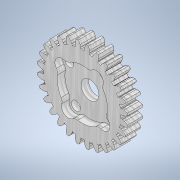
# Autodesk Inventor part: m1歯数28ギア5td6
Saved by Autodesk Inventor 2020.2 (Build 242310000, 310)
## iProperties
Created: 2020-02-29
Part Number: m1歯数28ギア5td6
Material: アルミニウム 7075
Document SubType Name: Modeling
Designer: aoyam
Density: 2.81 g/cm^3
Appearance: サテン - ブラシ仕上げ 重厚
Author: aoyam
Autodesk Inventor part; units mm, degrees
ref_plane "YZ Plane" through (0, 0, 0) normal (1, 0, 0) x (0, 1, 0)
ref_plane "XZ Plane" through (0, 0, 0) normal (0, 1, 0) x (-1, 0, 0)
ref_plane "XY Plane" through (0, 0, 0) normal (0, 0, 1) x (1, 0, 0)
sketch "スケッチ1" plane through (0, 0, 0) normal (0, 0, 1) x (1, 0, 0)
  arc A0 (-2.9821, 27.222) -> (-3.0107, 27.0374) centre (-1.7695, 26.9398) ccw
  arc A1 (-2.798, 27.798) -> (-2.9821, 27.222) centre (0.3539, 26.4732) ccw
  arc A2 (-2.2367, 28.835) -> (-2.798, 27.798) centre (2.6408, 25.5245) ccw
  arc A3 (-4.0943, 27.0374) -> (-4.1229, 27.222) centre (-5.3355, 26.9398) ccw
  arc A4 (-4.1229, 27.222) -> (-4.307, 27.798) centre (-7.4589, 26.4732) ccw
  arc A5 (-4.307, 27.798) -> (-4.8683, 28.835) centre (-9.7458, 25.5245) ccw
  arc A6 (-3.0274, 26.632) -> (-4.0776, 26.632) centre (-3.5525, 13.8928) ccw
  arc A7 (-4.8683, 28.835) -> (-5.5946, 28.7532) centre (-3.5525, 13.8928) ccw
  line L0 (-3.0274, 26.632) -> (-3.0107, 27.0374)
  line L1 (-4.0776, 26.632) -> (-4.0943, 27.0374)
  line L2 (-6.8991, 26.1958) -> (-7.0056, 26.5873)
  arc A8 (-7.0056, 26.5873) -> (-7.0746, 26.7609) centre (-8.194, 26.2159) ccw
  arc A9 (-7.0746, 26.7609) -> (-7.3822, 27.2815) centre (-10.1603, 25.2886) ccw
  arc A10 (-7.3822, 27.2815) -> (-8.1602, 28.1676) centre (-12.1788, 23.8547) ccw
  arc A11 (-8.1602, 28.1676) -> (-8.8502, 27.9262) centre (-3.5525, 13.8928) ccw
  arc A12 (-5.8753, 26.4295) -> (-6.8991, 26.1958) centre (-3.5525, 13.8928) ccw
  line L3 (-5.8753, 26.4295) -> (-5.9492, 26.8284)
  arc A13 (-5.9624, 27.0148) -> (-5.9492, 26.8284) centre (-4.7174, 27.0094) ccw
  arc A14 (-5.9111, 27.6173) -> (-5.9624, 27.0148) centre (-2.5434, 27.0271) ccw
  arc A15 (-5.5946, 28.7532) -> (-5.9111, 27.6173) centre (-0.1027, 26.611) ccw
  line L4 (-9.5529, 25.1426) -> (-9.7438, 25.5006)
  arc A16 (-9.7438, 25.5006) -> (-9.8497, 25.6546) centre (-10.8197, 24.8741) ccw
  arc A17 (-9.8497, 25.6546) -> (-10.2655, 26.0936) centre (-12.5304, 23.5325) ccw
  arc A18 (-10.2655, 26.0936) -> (-11.2211, 26.7844) centre (-14.1792, 21.6854) ccw
  arc A19 (-11.2211, 26.7844) -> (-11.84, 26.3955) centre (-3.5525, 13.8928) ccw
  arc A20 (-8.6067, 25.5983) -> (-9.5529, 25.1426) centre (-3.5525, 13.8928) ccw
  line L5 (-8.6067, 25.5983) -> (-8.7675, 25.9707)
  arc A21 (-8.8219, 26.1495) -> (-8.7675, 25.9707) centre (-7.6069, 26.4213) ccw
  arc A22 (-8.9059, 26.7483) -> (-8.8219, 26.1495) centre (-5.4914, 26.9223) ccw
  arc A23 (-8.8502, 27.9262) -> (-8.9059, 26.7483) centre (-3.0193, 27.0598) ccw
  line L6 (-11.9058, 23.5254) -> (-12.1716, 23.8319)
  arc A24 (-12.1716, 23.8319) -> (-12.309, 23.9584) centre (-13.0811, 22.9817) ccw
  arc A25 (-12.309, 23.9584) -> (-12.8121, 24.2939) centre (-14.4504, 21.293) ccw
  arc A26 (-12.8121, 24.2939) -> (-13.8975, 24.7547) centre (-15.6468, 19.1254) ccw
  arc A27 (-13.8975, 24.7547) -> (-14.4144, 24.2379) centre (-3.5525, 13.8928) ccw
  arc A28 (-11.0847, 24.1801) -> (-11.9058, 23.5254) centre (-3.5525, 13.8928) ccw
  line L7 (-11.0847, 24.1801) -> (-11.3244, 24.5075)
  arc A29 (-11.4171, 24.6697) -> (-11.3244, 24.5075) centre (-10.2931, 25.205) ccw
  arc A30 (-11.6323, 25.2347) -> (-11.4171, 24.6697) centre (-8.3421, 26.1642) ccw
  arc A31 (-11.84, 26.3955) -> (-11.6323, 25.2347) centre (-5.9626, 26.8483) ccw
  line L8 (-13.8398, 21.4251) -> (-14.1671, 21.6647)
  arc A32 (-14.1671, 21.6647) -> (-14.3293, 21.7575) centre (-14.8646, 20.6335) ccw
  arc A33 (-14.3293, 21.7575) -> (-14.8944, 21.9727) centre (-15.8238, 18.6824) ccw
  arc A34 (-14.8944, 21.9727) -> (-16.0551, 22.1804) centre (-16.5079, 16.3029) ccw
  arc A35 (-16.0551, 22.1804) -> (-16.444, 21.5615) centre (-3.5525, 13.8928) ccw
  arc A36 (-13.185, 22.2461) -> (-13.8398, 21.4251) centre (-3.5525, 13.8928) ccw
  line L9 (-13.185, 22.2461) -> (-13.4915, 22.5119)
  arc A37 (-13.618, 22.6494) -> (-13.4915, 22.5119) centre (-12.6413, 23.4214) ccw
  arc A38 (-13.9536, 23.1524) -> (-13.618, 22.6494) centre (-10.9526, 24.7907) ccw
  arc A39 (-14.4144, 24.2379) -> (-13.9536, 23.1524) centre (-8.785, 25.9872) ccw
  line L10 (-15.2579, 18.9471) -> (-15.6304, 19.1079)
  arc A40 (-15.6304, 19.1079) -> (-15.8092, 19.1623) centre (-16.0809, 17.9473) ccw
  arc A41 (-15.8092, 19.1623) -> (-16.4079, 19.2463) centre (-16.5819, 15.8317) ccw
  arc A42 (-16.4079, 19.2463) -> (-17.5858, 19.1905) centre (-16.7194, 13.3597) ccw
  arc A43 (-17.5858, 19.1905) -> (-17.8272, 18.5006) centre (-3.5525, 13.8928) ccw
  arc A44 (-14.8023, 19.8933) -> (-15.2579, 18.9471) centre (-3.5525, 13.8928) ccw
  line L11 (-14.8023, 19.8933) -> (-15.1602, 20.0842)
  arc A45 (-15.3142, 20.1901) -> (-15.1602, 20.0842) centre (-14.5337, 21.1601) ccw
  arc A46 (-15.7532, 20.6058) -> (-15.3142, 20.1901) centre (-13.1921, 22.8708) ccw
  arc A47 (-16.444, 21.5615) -> (-15.7532, 20.6058) centre (-11.3451, 24.5196) ccw
  line L12 (-16.0891, 16.2157) -> (-16.488, 16.2896)
  arc A48 (-16.488, 16.2896) -> (-16.6744, 16.3028) centre (-16.669, 15.0578) ccw
  arc A49 (-16.6744, 16.3028) -> (-17.2769, 16.2515) centre (-16.6867, 12.8838) ccw
  arc A50 (-17.2769, 16.2515) -> (-18.4128, 15.935) centre (-16.2707, 10.4431) ccw
  arc A51 (-18.4128, 15.935) -> (-18.4947, 15.2086) centre (-3.5525, 13.8928) ccw
  arc A52 (-15.8554, 17.2395) -> (-16.0891, 16.2157) centre (-3.5525, 13.8928) ccw
  line L13 (-15.8554, 17.2395) -> (-16.2469, 17.346)
  arc A53 (-16.4206, 17.415) -> (-16.2469, 17.346) centre (-15.8755, 18.5343) ccw
  arc A54 (-16.9411, 17.7226) -> (-16.4206, 17.415) centre (-14.9482, 20.5007) ccw
  arc A55 (-17.8272, 18.5006) -> (-16.9411, 17.7226) centre (-13.5144, 22.5192) ccw
  line L14 (-16.2917, 13.3678) -> (-16.697, 13.351)
  arc A56 (-16.697, 13.351) -> (-16.8817, 13.3225) centre (-16.5994, 12.1099) ccw
  arc A57 (-16.8817, 13.3225) -> (-17.4576, 13.1384) centre (-16.1329, 9.9864) ccw
  arc A58 (-17.4576, 13.1384) -> (-18.4947, 12.5771) centre (-15.1841, 7.6995) ccw
  arc A59 (-18.4947, 12.5771) -> (-18.4128, 11.8507) centre (-3.5525, 13.8928) ccw
  arc A60 (-16.2917, 14.4179) -> (-16.2917, 13.3678) centre (-3.5525, 13.8928) ccw
  line L15 (-16.2917, 14.4179) -> (-16.697, 14.4346)
  arc A61 (-16.8817, 14.4632) -> (-16.697, 14.4346) centre (-16.5994, 15.6758) ccw
  arc A62 (-17.4576, 14.6473) -> (-16.8817, 14.4632) centre (-16.1329, 17.7992) ccw
  arc A63 (-18.4947, 15.2086) -> (-17.4576, 14.6473) centre (-15.1841, 20.0862) ccw
  line L16 (-15.8554, 10.5462) -> (-16.2469, 10.4397)
  arc A64 (-16.2469, 10.4397) -> (-16.4206, 10.3707) centre (-15.8755, 9.2514) ccw
  arc A65 (-16.4206, 10.3707) -> (-16.9411, 10.0631) centre (-14.9482, 7.285) ccw
  arc A66 (-16.9411, 10.0631) -> (-17.8272, 9.2851) centre (-13.5144, 5.2665) ccw
  arc A67 (-17.8272, 9.2851) -> (-17.5858, 8.5952) centre (-3.5525, 13.8928) ccw
  arc A68 (-16.0891, 11.57) -> (-15.8554, 10.5462) centre (-3.5525, 13.8928) ccw
  line L17 (-16.0891, 11.57) -> (-16.488, 11.4961)
  arc A69 (-16.6744, 11.4829) -> (-16.488, 11.4961) centre (-16.669, 12.7279) ccw
  arc A70 (-17.2769, 11.5342) -> (-16.6744, 11.4829) centre (-16.6867, 14.9019) ccw
  arc A71 (-18.4128, 11.8507) -> (-17.2769, 11.5342) centre (-16.2707, 17.3426) ccw
  line L18 (-14.8023, 7.8924) -> (-15.1602, 7.7015)
  arc A72 (-15.1602, 7.7015) -> (-15.3142, 7.5956) centre (-14.5337, 6.6256) ccw
  arc A73 (-15.3142, 7.5956) -> (-15.7532, 7.1799) centre (-13.1921, 4.9149) ccw
  arc A74 (-15.7532, 7.1799) -> (-16.444, 6.2242) centre (-11.3451, 3.2661) ccw
  arc A75 (-16.444, 6.2242) -> (-16.0551, 5.6053) centre (-3.5525, 13.8928) ccw
  arc A76 (-15.2579, 8.8386) -> (-14.8023, 7.8924) centre (-3.5525, 13.8928) ccw
  line L19 (-15.2579, 8.8386) -> (-15.6304, 8.6778)
  arc A77 (-15.8092, 8.6234) -> (-15.6304, 8.6778) centre (-16.0809, 9.8384) ccw
  arc A78 (-16.4079, 8.5394) -> (-15.8092, 8.6234) centre (-16.5819, 11.954) ccw
  arc A79 (-17.5858, 8.5952) -> (-16.4079, 8.5394) centre (-16.7194, 14.426) ccw
  line L20 (-13.185, 5.5396) -> (-13.4915, 5.2738)
  arc A80 (-13.4915, 5.2738) -> (-13.618, 5.1363) centre (-12.6413, 4.3642) ccw
  arc A81 (-13.618, 5.1363) -> (-13.9536, 4.6333) centre (-10.9526, 2.995) ccw
  arc A82 (-13.9536, 4.6333) -> (-14.4144, 3.5478) centre (-8.785, 1.7985) ccw
  arc A83 (-14.4144, 3.5478) -> (-13.8975, 3.031) centre (-3.5525, 13.8928) ccw
  arc A84 (-13.8398, 6.3606) -> (-13.185, 5.5396) centre (-3.5525, 13.8928) ccw
  line L21 (-13.8398, 6.3606) -> (-14.1671, 6.121)
  arc A85 (-14.3293, 6.0282) -> (-14.1671, 6.121) centre (-14.8646, 7.1522) ccw
  arc A86 (-14.8944, 5.813) -> (-14.3293, 6.0282) centre (-15.8238, 9.1033) ccw
  arc A87 (-16.0551, 5.6053) -> (-14.8944, 5.813) centre (-16.5079, 11.4827) ccw
  line L22 (-11.0847, 3.6056) -> (-11.3244, 3.2782)
  arc A88 (-11.3244, 3.2782) -> (-11.4171, 3.116) centre (-10.2931, 2.5807) ccw
  arc A89 (-11.4171, 3.116) -> (-11.6323, 2.551) centre (-8.3421, 1.6215) ccw
  arc A90 (-11.6323, 2.551) -> (-11.84, 1.3902) centre (-5.9626, 0.9374) ccw
  arc A91 (-11.84, 1.3902) -> (-11.2211, 1.0013) centre (-3.5525, 13.8928) ccw
  arc A92 (-11.9058, 4.2603) -> (-11.0847, 3.6056) centre (-3.5525, 13.8928) ccw
  line L23 (-11.9058, 4.2603) -> (-12.1716, 3.9538)
  arc A93 (-12.309, 3.8273) -> (-12.1716, 3.9538) centre (-13.0811, 4.804) ccw
  arc A94 (-12.8121, 3.4918) -> (-12.309, 3.8273) centre (-14.4504, 6.4927) ccw
  arc A95 (-13.8975, 3.031) -> (-12.8121, 3.4918) centre (-15.6468, 8.6603) ccw
  line L24 (-8.6067, 2.1874) -> (-8.7675, 1.815)
  arc A96 (-8.7675, 1.815) -> (-8.8219, 1.6362) centre (-7.6069, 1.3644) ccw
  arc A97 (-8.8219, 1.6362) -> (-8.9059, 1.0374) centre (-5.4914, 0.8634) ccw
  arc A98 (-8.9059, 1.0374) -> (-8.8502, -0.1405) centre (-3.0193, 0.7259) ccw
  arc A99 (-8.8502, -0.1405) -> (-8.1602, -0.3819) centre (-3.5525, 13.8928) ccw
  arc A100 (-9.5529, 2.6431) -> (-8.6067, 2.1874) centre (-3.5525, 13.8928) ccw
  line L25 (-9.5529, 2.6431) -> (-9.7438, 2.2851)
  arc A101 (-9.8497, 2.1311) -> (-9.7438, 2.2851) centre (-10.8197, 2.9116) ccw
  arc A102 (-10.2655, 1.6921) -> (-9.8497, 2.1311) centre (-12.5304, 4.2532) ccw
  arc A103 (-11.2211, 1.0013) -> (-10.2655, 1.6921) centre (-14.1792, 6.1003) ccw
  line L26 (-5.8753, 1.3562) -> (-5.9492, 0.9573)
  arc A104 (-5.9492, 0.9573) -> (-5.9624, 0.7709) centre (-4.7174, 0.7763) ccw
  arc A105 (-5.9624, 0.7709) -> (-5.9111, 0.1684) centre (-2.5434, 0.7586) ccw
  arc A106 (-5.9111, 0.1684) -> (-5.5946, -0.9675) centre (-0.1027, 1.1747) ccw
  arc A107 (-5.5946, -0.9675) -> (-4.8683, -1.0493) centre (-3.5525, 13.8928) ccw
  arc A108 (-6.8991, 1.5899) -> (-5.8753, 1.3562) centre (-3.5525, 13.8928) ccw
  line L27 (-6.8991, 1.5899) -> (-7.0056, 1.1984)
  arc A109 (-7.0746, 1.0248) -> (-7.0056, 1.1984) centre (-8.194, 1.5698) ccw
  arc A110 (-7.3822, 0.5042) -> (-7.0746, 1.0248) centre (-10.1603, 2.4971) ccw
  arc A111 (-8.1602, -0.3819) -> (-7.3822, 0.5042) centre (-12.1788, 3.931) ccw
  line L28 (-3.0274, 1.1537) -> (-3.0107, 0.7483)
  arc A112 (-3.0107, 0.7483) -> (-2.9821, 0.5637) centre (-1.7695, 0.8459) ccw
  arc A113 (-2.9821, 0.5637) -> (-2.798, -0.0123) centre (0.3539, 1.3125) ccw
  arc A114 (-2.798, -0.0123) -> (-2.2367, -1.0493) centre (2.6408, 2.2612) ccw
  arc A115 (-2.2367, -1.0493) -> (-1.5103, -0.9675) centre (-3.5525, 13.8928) ccw
  arc A116 (-4.0776, 1.1537) -> (-3.0274, 1.1537) centre (-3.5525, 13.8928) ccw
  line L29 (-4.0776, 1.1537) -> (-4.0943, 0.7483)
  arc A117 (-4.1229, 0.5637) -> (-4.0943, 0.7483) centre (-5.3355, 0.8459) ccw
  arc A118 (-4.307, -0.0123) -> (-4.1229, 0.5637) centre (-7.4589, 1.3125) ccw
  arc A119 (-4.8683, -1.0493) -> (-4.307, -0.0123) centre (-9.7458, 2.2612) ccw
  line L30 (-0.2058, 1.5899) -> (-0.0993, 1.1984)
  arc A120 (-0.0993, 1.1984) -> (-0.0304, 1.0248) centre (1.089, 1.5698) ccw
  arc A121 (-0.0304, 1.0248) -> (0.2773, 0.5042) centre (3.0554, 2.4971) ccw
  arc A122 (0.2773, 0.5042) -> (1.0553, -0.3819) centre (5.0738, 3.931) ccw
  arc A123 (1.0553, -0.3819) -> (1.7452, -0.1405) centre (-3.5525, 13.8928) ccw
  arc A124 (-1.2297, 1.3562) -> (-0.2058, 1.5899) centre (-3.5525, 13.8928) ccw
  line L31 (-1.2297, 1.3562) -> (-1.1558, 0.9573)
  arc A125 (-1.1425, 0.7709) -> (-1.1558, 0.9573) centre (-2.3875, 0.7763) ccw
  arc A126 (-1.1938, 0.1684) -> (-1.1425, 0.7709) centre (-4.5615, 0.7586) ccw
  arc A127 (-1.5103, -0.9675) -> (-1.1938, 0.1684) centre (-7.0022, 1.1747) ccw
  line L32 (2.4479, 2.6431) -> (2.6389, 2.2851)
  arc A128 (2.6389, 2.2851) -> (2.7447, 2.1311) centre (3.7148, 2.9116) ccw
  arc A129 (2.7447, 2.1311) -> (3.1605, 1.6921) centre (5.4255, 4.2532) ccw
  arc A130 (3.1605, 1.6921) -> (4.1162, 1.0013) centre (7.0743, 6.1003) ccw
  arc A131 (4.1162, 1.0013) -> (4.7351, 1.3902) centre (-3.5525, 13.8928) ccw
  arc A132 (1.5018, 2.1874) -> (2.4479, 2.6431) centre (-3.5525, 13.8928) ccw
  line L33 (1.5018, 2.1874) -> (1.6626, 1.815)
  arc A133 (1.7169, 1.6362) -> (1.6626, 1.815) centre (0.502, 1.3644) ccw
  arc A134 (1.801, 1.0374) -> (1.7169, 1.6362) centre (-1.6136, 0.8634) ccw
  arc A135 (1.7452, -0.1405) -> (1.801, 1.0374) centre (-4.0857, 0.7259) ccw
  line L34 (4.8008, 4.2603) -> (5.0666, 3.9538)
  arc A136 (5.0666, 3.9538) -> (5.2041, 3.8273) centre (5.9761, 4.804) ccw
  arc A137 (5.2041, 3.8273) -> (5.7071, 3.4918) centre (7.3454, 6.4927) ccw
  arc A138 (5.7071, 3.4918) -> (6.7925, 3.031) centre (8.5419, 8.6603) ccw
  arc A139 (6.7925, 3.031) -> (7.3094, 3.5478) centre (-3.5525, 13.8928) ccw
  arc A140 (3.9797, 3.6056) -> (4.8008, 4.2603) centre (-3.5525, 13.8928) ccw
  line L35 (3.9797, 3.6056) -> (4.2194, 3.2782)
  arc A141 (4.3122, 3.116) -> (4.2194, 3.2782) centre (3.1881, 2.5807) ccw
  arc A142 (4.5274, 2.551) -> (4.3122, 3.116) centre (1.2371, 1.6215) ccw
  arc A143 (4.7351, 1.3902) -> (4.5274, 2.551) centre (-1.1424, 0.9374) ccw
  line L36 (6.7348, 6.3606) -> (7.0621, 6.121)
  arc A144 (7.0621, 6.121) -> (7.2243, 6.0282) centre (7.7597, 7.1522) ccw
  arc A145 (7.2243, 6.0282) -> (7.7894, 5.813) centre (8.7189, 9.1033) ccw
  arc A146 (7.7894, 5.813) -> (8.9502, 5.6053) centre (9.403, 11.4827) ccw
  arc A147 (8.9502, 5.6053) -> (9.3391, 6.2242) centre (-3.5525, 13.8928) ccw
  arc A148 (6.08, 5.5396) -> (6.7348, 6.3606) centre (-3.5525, 13.8928) ccw
  line L37 (6.08, 5.5396) -> (6.3865, 5.2738)
  arc A149 (6.5131, 5.1363) -> (6.3865, 5.2738) centre (5.5363, 4.3642) ccw
  arc A150 (6.8486, 4.6333) -> (6.5131, 5.1363) centre (3.8477, 2.995) ccw
  arc A151 (7.3094, 3.5478) -> (6.8486, 4.6333) centre (1.6801, 1.7985) ccw
  line L38 (8.153, 8.8386) -> (8.5254, 8.6778)
  arc A152 (8.5254, 8.6778) -> (8.7042, 8.6234) centre (8.976, 9.8384) ccw
  arc A153 (8.7042, 8.6234) -> (9.303, 8.5394) centre (9.477, 11.954) ccw
  arc A154 (9.303, 8.5394) -> (10.4809, 8.5952) centre (9.6145, 14.426) ccw
  arc A155 (10.4809, 8.5952) -> (10.7223, 9.2851) centre (-3.5525, 13.8928) ccw
  arc A156 (7.6973, 7.8924) -> (8.153, 8.8386) centre (-3.5525, 13.8928) ccw
  line L39 (7.6973, 7.8924) -> (8.0553, 7.7015)
  arc A157 (8.2092, 7.5956) -> (8.0553, 7.7015) centre (7.4288, 6.6256) ccw
  arc A158 (8.6483, 7.1799) -> (8.2092, 7.5956) centre (6.0871, 4.9149) ccw
  arc A159 (9.3391, 6.2242) -> (8.6483, 7.1799) centre (4.2401, 3.2661) ccw
  line L40 (8.9841, 11.57) -> (9.3831, 11.4961)
  arc A160 (9.3831, 11.4961) -> (9.5694, 11.4829) centre (9.5641, 12.7279) ccw
  arc A161 (9.5694, 11.4829) -> (10.1719, 11.5342) centre (9.5817, 14.9019) ccw
  arc A162 (10.1719, 11.5342) -> (11.3079, 11.8507) centre (9.1657, 17.3426) ccw
  arc A163 (11.3079, 11.8507) -> (11.3897, 12.5771) centre (-3.5525, 13.8928) ccw
  arc A164 (8.7505, 10.5462) -> (8.9841, 11.57) centre (-3.5525, 13.8928) ccw
  line L41 (8.7505, 10.5462) -> (9.1419, 10.4397)
  arc A165 (9.3156, 10.3707) -> (9.1419, 10.4397) centre (8.7706, 9.2514) ccw
  arc A166 (9.8362, 10.0631) -> (9.3156, 10.3707) centre (7.8432, 7.285) ccw
  arc A167 (10.7223, 9.2851) -> (9.8362, 10.0631) centre (6.4094, 5.2665) ccw
  line L42 (9.1867, 14.4179) -> (9.5921, 14.4346)
  arc A168 (9.5921, 14.4346) -> (9.7767, 14.4632) centre (9.4944, 15.6758) ccw
  arc A169 (9.7767, 14.4632) -> (10.3527, 14.6473) centre (9.0279, 17.7992) ccw
  arc A170 (10.3527, 14.6473) -> (11.3897, 15.2086) centre (8.0792, 20.0862) ccw
  arc A171 (11.3897, 15.2086) -> (11.3079, 15.935) centre (-3.5525, 13.8928) ccw
  arc A172 (9.1867, 13.3678) -> (9.1867, 14.4179) centre (-3.5525, 13.8928) ccw
  line L43 (9.1867, 13.3678) -> (9.5921, 13.351)
  arc A173 (9.7767, 13.3225) -> (9.5921, 13.351) centre (9.4944, 12.1099) ccw
  arc A174 (10.3527, 13.1384) -> (9.7767, 13.3225) centre (9.0279, 9.9864) ccw
  arc A175 (11.3897, 12.5771) -> (10.3527, 13.1384) centre (8.0792, 7.6995) ccw
  line L44 (8.7505, 17.2395) -> (9.1419, 17.346)
  arc A176 (9.1419, 17.346) -> (9.3156, 17.415) centre (8.7706, 18.5343) ccw
  arc A177 (9.3156, 17.415) -> (9.8362, 17.7226) centre (7.8432, 20.5007) ccw
  arc A178 (9.8362, 17.7226) -> (10.7223, 18.5006) centre (6.4094, 22.5192) ccw
  arc A179 (10.7223, 18.5006) -> (10.4809, 19.1905) centre (-3.5525, 13.8928) ccw
  arc A180 (8.9841, 16.2157) -> (8.7505, 17.2395) centre (-3.5525, 13.8928) ccw
  line L45 (8.9841, 16.2157) -> (9.3831, 16.2896)
  arc A181 (9.5694, 16.3028) -> (9.3831, 16.2896) centre (9.5641, 15.0578) ccw
  arc A182 (10.1719, 16.2515) -> (9.5694, 16.3028) centre (9.5817, 12.8838) ccw
  arc A183 (11.3079, 15.935) -> (10.1719, 16.2515) centre (9.1657, 10.4431) ccw
  line L46 (7.6973, 19.8933) -> (8.0553, 20.0842)
  arc A184 (8.0553, 20.0842) -> (8.2092, 20.1901) centre (7.4288, 21.1601) ccw
  arc A185 (8.2092, 20.1901) -> (8.6483, 20.6058) centre (6.0871, 22.8708) ccw
  arc A186 (8.6483, 20.6058) -> (9.3391, 21.5615) centre (4.2401, 24.5196) ccw
  arc A187 (9.3391, 21.5615) -> (8.9502, 22.1804) centre (-3.5525, 13.8928) ccw
  arc A188 (8.153, 18.9471) -> (7.6973, 19.8933) centre (-3.5525, 13.8928) ccw
  line L47 (8.153, 18.9471) -> (8.5254, 19.1079)
  arc A189 (8.7042, 19.1623) -> (8.5254, 19.1079) centre (8.976, 17.9473) ccw
  arc A190 (9.303, 19.2463) -> (8.7042, 19.1623) centre (9.477, 15.8317) ccw
  arc A191 (10.4809, 19.1905) -> (9.303, 19.2463) centre (9.6145, 13.3597) ccw
  line L48 (6.08, 22.2461) -> (6.3865, 22.5119)
  arc A192 (6.3865, 22.5119) -> (6.5131, 22.6494) centre (5.5363, 23.4214) ccw
  arc A193 (6.5131, 22.6494) -> (6.8486, 23.1524) centre (3.8477, 24.7907) ccw
  arc A194 (6.8486, 23.1524) -> (7.3094, 24.2379) centre (1.6801, 25.9872) ccw
  arc A195 (7.3094, 24.2379) -> (6.7925, 24.7547) centre (-3.5525, 13.8928) ccw
  arc A196 (6.7348, 21.4251) -> (6.08, 22.2461) centre (-3.5525, 13.8928) ccw
  line L49 (6.7348, 21.4251) -> (7.0621, 21.6647)
  arc A197 (7.2243, 21.7575) -> (7.0621, 21.6647) centre (7.7597, 20.6335) ccw
  arc A198 (7.7894, 21.9727) -> (7.2243, 21.7575) centre (8.7189, 18.6824) ccw
  arc A199 (8.9502, 22.1804) -> (7.7894, 21.9727) centre (9.403, 16.3029) ccw
  line L50 (3.9797, 24.1801) -> (4.2194, 24.5075)
  arc A200 (4.2194, 24.5075) -> (4.3122, 24.6697) centre (3.1881, 25.205) ccw
  arc A201 (4.3122, 24.6697) -> (4.5274, 25.2347) centre (1.2371, 26.1642) ccw
  arc A202 (4.5274, 25.2347) -> (4.7351, 26.3955) centre (-1.1424, 26.8483) ccw
  arc A203 (4.7351, 26.3955) -> (4.1162, 26.7844) centre (-3.5525, 13.8928) ccw
  arc A204 (4.8008, 23.5254) -> (3.9797, 24.1801) centre (-3.5525, 13.8928) ccw
  line L51 (4.8008, 23.5254) -> (5.0666, 23.8319)
  arc A205 (5.2041, 23.9584) -> (5.0666, 23.8319) centre (5.9761, 22.9817) ccw
  arc A206 (5.7071, 24.2939) -> (5.2041, 23.9584) centre (7.3454, 21.293) ccw
  arc A207 (6.7925, 24.7547) -> (5.7071, 24.2939) centre (8.5419, 19.1254) ccw
  line L52 (1.5018, 25.5983) -> (1.6626, 25.9707)
  arc A208 (1.6626, 25.9707) -> (1.7169, 26.1495) centre (0.502, 26.4213) ccw
  arc A209 (1.7169, 26.1495) -> (1.801, 26.7483) centre (-1.6136, 26.9223) ccw
  arc A210 (1.801, 26.7483) -> (1.7452, 27.9262) centre (-4.0857, 27.0598) ccw
  arc A211 (1.7452, 27.9262) -> (1.0553, 28.1676) centre (-3.5525, 13.8928) ccw
  arc A212 (2.4479, 25.1426) -> (1.5018, 25.5983) centre (-3.5525, 13.8928) ccw
  line L53 (2.4479, 25.1426) -> (2.6389, 25.5006)
  arc A213 (2.7447, 25.6546) -> (2.6389, 25.5006) centre (3.7148, 24.8741) ccw
  arc A214 (3.1605, 26.0936) -> (2.7447, 25.6546) centre (5.4255, 23.5325) ccw
  arc A215 (4.1162, 26.7844) -> (3.1605, 26.0936) centre (7.0743, 21.6854) ccw
  line L54 (-1.2297, 26.4295) -> (-1.1558, 26.8284)
  arc A216 (-1.1558, 26.8284) -> (-1.1425, 27.0148) centre (-2.3875, 27.0094) ccw
  arc A217 (-1.1425, 27.0148) -> (-1.1938, 27.6173) centre (-4.5615, 27.0271) ccw
  arc A218 (-1.1938, 27.6173) -> (-1.5103, 28.7532) centre (-7.0022, 26.611) ccw
  arc A219 (-1.5103, 28.7532) -> (-2.2367, 28.835) centre (-3.5525, 13.8928) ccw
  arc A220 (-0.2058, 26.1958) -> (-1.2297, 26.4295) centre (-3.5525, 13.8928) ccw
  line L55 (-0.2058, 26.1958) -> (-0.0993, 26.5873)
  arc A221 (-0.0304, 26.7609) -> (-0.0993, 26.5873) centre (1.089, 26.2159) ccw
  arc A222 (0.2773, 27.2815) -> (-0.0304, 26.7609) centre (3.0554, 25.2886) ccw
  arc A223 (1.0553, 28.1676) -> (0.2773, 27.2815) centre (5.0738, 23.8547) ccw
  circle A224 centre (-3.5525, 13.8928) radius 2.99
  circle A225 centre (-3.5525, 13.8928) radius 8.25
  circle A226 centre (-10.3702, 18.5385) radius 1.5
  circle A227 centre (-8.1981, 7.0752) radius 1.5
  circle A228 centre (3.2652, 9.2472) radius 1.5
  circle A229 centre (1.0931, 20.7105) radius 1.5
  circle A230 centre (-3.5525, 13.8928) radius 8.3
  circle A231 centre (3.2652, 9.2472) radius 3.5
  circle A232 centre (1.0931, 20.7105) radius 3.5
  circle A233 centre (-10.3702, 18.5385) radius 3.5
  circle A234 centre (-8.1981, 7.0752) radius 3.5
  circle A235 centre (-10.3702, 18.5385) radius 2.25
  circle A236 centre (-10.3702, 18.5385) radius 2.3
  circle A237 centre (-8.1981, 7.0752) radius 2.3
  circle A238 centre (-8.1981, 7.0752) radius 2.25
  circle A239 centre (3.2652, 9.2472) radius 2.3
  circle A240 centre (3.2652, 9.2472) radius 2.25
  circle A241 centre (1.0931, 20.7105) radius 2.3
  circle A242 centre (1.0931, 20.7105) radius 2.25
  point P0 (0, 0)
  point P1 (-3.0274, 26.632)
  point P2 (-4.0776, 26.632)
  point P3 (-3.0081, 17.5003)
  point P4 (-4.1229, 27.222)
  point P5 (-4.307, 27.798)
  point P6 (-4.8683, 28.835)
  point P7 (-5.5946, 28.7532)
  point P8 (-5.9111, 27.6173)
  point P9 (-5.9624, 27.0148)
  point P10 (-4.863, 17.2913)
  point P11 (-5.8753, 26.4295)
  point P12 (-6.8991, 26.1958)
  point P13 (-5.9194, 17.0502)
  point P14 (-7.0746, 26.7609)
  point P15 (-7.3822, 27.2815)
  point P16 (-8.1602, 28.1676)
  point P17 (-8.8502, 27.9262)
  point P18 (-8.9059, 26.7483)
  point P19 (-8.8219, 26.1495)
  point P20 (-7.6813, 16.4337)
  point P21 (-8.6067, 25.5983)
  point P22 (-9.5529, 25.1426)
  point P23 (-8.6576, 15.9635)
  point P24 (-9.8497, 25.6546)
  point P25 (-10.2655, 26.0936)
  point P26 (-11.2211, 26.7844)
  point P27 (-11.84, 26.3955)
  point P28 (-11.6323, 25.2347)
  point P29 (-11.4171, 24.6697)
  point P30 (-10.2382, 14.9704)
  point P31 (-11.0847, 24.1801)
  point P32 (-11.9058, 23.5254)
  point P33 (-11.0854, 14.2948)
  point P34 (-12.309, 23.9584)
  point P35 (-12.8121, 24.2939)
  point P36 (-13.8975, 24.7547)
  point P37 (-14.4144, 24.2379)
  point P38 (-13.618, 22.6494)
  point P39 (-12.4053, 12.9749)
  point P40 (-13.185, 22.2461)
  point P41 (-13.8398, 21.4251)
  point P42 (-13.0809, 12.1277)
  point P43 (-14.3293, 21.7575)
  point P44 (-16.0551, 22.1804)
  point P45 (-16.444, 21.5615)
  point P46 (-15.7532, 20.6058)
  point P47 (-15.3142, 20.1901)
  point P48 (-14.074, 10.5471)
  point P49 (-14.8023, 19.8933)
  point P50 (-15.2579, 18.9471)
  point P51 (-14.5442, 9.5709)
  point P52 (-17.5858, 19.1905)
  point P53 (-17.8272, 18.5006)
  point P54 (-16.9411, 17.7226)
  point P55 (-15.1607, 7.809)
  point P56 (-15.8554, 17.2395)
  point P57 (-16.0891, 16.2157)
  point P58 (-15.4018, 6.7525)
  point P59 (-18.4128, 15.935)
  point P60 (-18.4947, 15.2086)
  point P61 (-17.4576, 14.6473)
  point P62 (-15.6108, 4.8976)
  point P63 (-16.2917, 14.4179)
  point P64 (-16.2917, 13.3678)
  point P65 (-15.6108, 3.814)
  point P66 (-17.4576, 13.1384)
  point P67 (-18.4947, 12.5771)
  point P68 (-18.4128, 11.8507)
  point P69 (-15.4018, 1.9591)
  point P70 (-16.0891, 11.57)
  point P71 (-15.8554, 10.5462)
  point P72 (-15.1607, 0.9026)
  point P73 (-17.8272, 9.2851)
  point P74 (-17.5858, 8.5952)
  point P75 (-16.4079, 8.5394)
  point P76 (-14.5442, -0.8593)
  point P77 (-15.2579, 8.8386)
  point P78 (-14.8023, 7.8924)
  point P79 (-14.074, -1.8355)
  point P80 (-15.7532, 7.1799)
  point P81 (-16.444, 6.2242)
  point P82 (-16.0551, 5.6053)
  point P83 (-14.8944, 5.813)
  point P84 (-14.3293, 6.0282)
  point P85 (-13.0809, -3.4161)
  point P86 (-13.8398, 6.3606)
  point P87 (-13.185, 5.5396)
  point P88 (-12.4053, -4.2633)
  point P89 (-13.618, 5.1363)
  point P90 (-13.9536, 4.6333)
  point P91 (-14.4144, 3.5478)
  point P92 (-13.8975, 3.031)
  point P93 (-12.8121, 3.4918)
  point P94 (-12.309, 3.8273)
  point P95 (-11.0854, -5.5832)
  point P96 (-11.9058, 4.2603)
  point P97 (-11.0847, 3.6056)
  point P98 (-10.2382, -6.2588)
  point P99 (-11.4171, 3.116)
  point P100 (-11.6323, 2.551)
  point P101 (-11.84, 1.3902)
  point P102 (-11.2211, 1.0013)
  point P103 (-10.2655, 1.6921)
  point P104 (-9.8497, 2.1311)
  point P105 (-8.6576, -7.2519)
  point P106 (-9.5529, 2.6431)
  point P107 (-8.6067, 2.1874)
  point P108 (-7.6813, -7.7221)
  point P109 (-8.9059, 1.0374)
  point P110 (-8.8502, -0.1405)
  point P111 (-8.1602, -0.3819)
  point P112 (-7.3822, 0.5042)
  point P113 (-7.0746, 1.0248)
  point P114 (-5.9194, -8.3386)
  point P115 (-6.8991, 1.5899)
  point P116 (-5.8753, 1.3562)
  point P117 (-4.863, -8.5797)
  point P118 (-5.9624, 0.7709)
  point P119 (-5.9111, 0.1684)
  point P120 (-5.5946, -0.9675)
  point P121 (-4.8683, -1.0493)
  point P122 (-4.307, -0.0123)
  point P123 (-4.1229, 0.5637)
  point P124 (-3.0081, -8.7887)
  point P125 (-4.0776, 1.1537)
  point P126 (-3.0274, 1.1537)
  point P127 (-1.9245, -8.7887)
  point P128 (-2.9821, 0.5637)
  point P129 (-2.798, -0.0123)
  point P130 (-2.2367, -1.0493)
  point P131 (-1.5103, -0.9675)
  point P132 (-1.1938, 0.1684)
  point P133 (-1.1425, 0.7709)
  point P134 (-0.0696, -8.5797)
  point P135 (-1.2297, 1.3562)
  point P136 (-0.2058, 1.5899)
  point P137 (0.9869, -8.3386)
  point P138 (-0.0304, 1.0248)
  point P139 (0.2773, 0.5042)
  point P140 (1.0553, -0.3819)
  point P141 (1.7452, -0.1405)
  point P142 (1.801, 1.0374)
  point P143 (2.8031, -7.9009)
  point P144 (2.7488, -7.7221)
  point P145 (1.5018, 2.1874)
  point P146 (2.4479, 2.6431)
  point P147 (3.7251, -7.2519)
  point P148 (2.7447, 2.1311)
  point P149 (3.1605, 1.6921)
  point P150 (4.1162, 1.0013)
  point P151 (4.7351, 1.3902)
  point P152 (4.5274, 2.551)
  point P153 (4.3122, 3.116)
  point P154 (5.3056, -6.2588)
  point P155 (3.9797, 3.6056)
  point P156 (4.8008, 4.2603)
  point P157 (6.1528, -5.5832)
  point P158 (5.2041, 3.8273)
  point P159 (5.7071, 3.4918)
  point P160 (6.7925, 3.031)
  point P161 (7.3094, 3.5478)
  point P162 (6.8486, 4.6333)
  point P163 (6.5131, 5.1363)
  point P164 (7.4727, -4.2633)
  point P165 (6.08, 5.5396)
  point P166 (6.7348, 6.3606)
  point P167 (8.1483, -3.4161)
  point P168 (7.2243, 6.0282)
  point P169 (7.7894, 5.813)
  point P170 (8.9502, 5.6053)
  point P171 (9.3391, 6.2242)
  point P172 (8.6483, 7.1799)
  point P173 (8.2092, 7.5956)
  point P174 (9.1414, -1.8355)
  point P175 (7.6973, 7.8924)
  point P176 (8.153, 8.8386)
  point P177 (9.6116, -0.8593)
  point P178 (8.7042, 8.6234)
  point P179 (9.303, 8.5394)
  point P180 (10.4809, 8.5952)
  point P181 (10.7223, 9.2851)
  point P182 (9.8362, 10.0631)
  point P183 (10.2281, 0.9026)
  point P184 (8.7505, 10.5462)
  point P185 (8.9841, 11.57)
  point P186 (10.4692, 1.9591)
  point P187 (10.1719, 11.5342)
  point P188 (11.3079, 11.8507)
  point P189 (11.3897, 12.5771)
  point P190 (10.3527, 13.1384)
  point P191 (10.6782, 3.814)
  point P192 (9.1867, 13.3678)
  point P193 (9.1867, 14.4179)
  point P194 (10.6782, 4.8976)
  point P195 (9.7767, 14.4632)
  point P196 (10.3527, 14.6473)
  point P197 (11.3897, 15.2086)
  point P198 (11.3079, 15.935)
  point P199 (9.5694, 16.3028)
  dimension "d2" = 360
  dimension "d6" = 5.98
  dimension "d8" = 3
  dimension "d11" = 360
  dimension "d18" = 0.05
  dimension "d26" = 7
  dimension "d29" = 360
  dimension "d33" = 4.5
  dimension "d34" = 0.05
  dimension "d37" = 360
  constraints: 448 point on circle, 242 centre point, 112 end point, 5 coincident, 1097 other
  measures "d6" diameter of A224
  measures "d8" diameter of A226
  measures "d26" diameter of A231
  measures "d33" diameter of A235
  measures "d34" radial gap between concentric circles of A235 A236
extrude "押し出し1" add sketch "スケッチ1" along normal blind 5 contours A1 A2 A219 A218 A217 A216 L54 A220 L55 A221 A222 A223 A211 A210 A209 A208 L52 A212 L53 A213 A214 A215 A203 A202 A201 A200 L50 A204 L51 A205 A206 A207 A195 A194 A193 A192 L48 A196 L49 A197 A198 A199 A187 A186 A185 A184 L46 A188 L47 A189 A190 A191 A179 A178 A177 A176 L44 A180 L45 A181 A182 A183 A171 A170 A169 A168 L42 A172 L43 A173 A174 A175 A163 A162 A161 A160 L40 A164 L41 A165 A166 A167 A155 A154 A153 A152 L38 A156 L39 A157 A158 A159 A147 A146 A145 A144 L36 A148 L37 A149 A150 A151 A139 A138 A137 A136 L34 A140 L35 A141 A142 A143 A131 A130 A129 A128 L32 A132 L33 A133 A134 A135 A123 A122 A121 A120 L30 A124 L31 A125 A126 A127 A115 A114 A113 A112 L28 A116 L29 A117 A118 A119 A107 A106 A105 A104 L26 A108 L27 A109 A110 A111 A99 A98 A97 A96 L24 A100 L25 A101 A102 A103 A91 A90 A89 A88 L22 A92 L23 A93 A94 A95 A83 A82 A81 A80 L20 A84 L21 A85 A86 A87 A75 A74 A73 A72 L18 A76 L19 A77 A78 A79 A67 A66 A65 A64 L16 A68 L17 A69 A70 A71 A59 A58 A57 A56 L14 A60 L15 A61 A62 A63 A51 A50 A49 A48 L12 A52 L13 A53 A54 A55 A43 A42 A41 A40 L10 A44 L11 A45 A46 A47 A35 A34 A33 A32 L8 A36 L9 A37 A38 A39 A27 A26 A25 A24 L6 A28 L7 A29 A30 A31 A19 A18 A17 A16 L4 A20 L5 A21 A22 A23 A11 A10 A9 A8 L2 A12 L3 A13 A14 A15 A7 A5 A4 A3 L1 A6 L0 A0 | A230 A241 A232 | A231 A230 A239 | A230 A236 A233 | A234 A230 A237
extrude "押し出し2" add sketch "スケッチ1" along normal blind 2.5 contours A225 A231 A234 A233 A232 | A225 A232 A230 A231 | A232 A225 A241 | A225 A241 A230 A232 | A231 A230 A239 A225 | A225 A239 A231 | A241 A225 A242 | A225 A242 A230 A241 | A232 A230 A241 A225 | A225 A233 A230 A232 | A239 A230 A240 A225 | A225 A240 A239 | A231 A230 A234 A225 | A225 A239 A230 A231 | A242 A225 A229 | A225 A229 A230 A242 | A241 A230 A242 A225 | A230 A242 A241 | A233 A225 A236 | A225 A236 A230 A233 | A240 A230 A228 A225 | A225 A228 A240 | A239 A230 A240 | A225 A240 A230 A239 | A234 A230 A237 A225 | A225 A237 A234 | A242 A230 A229 A225 | A230 A229 A242 | A236 A225 A235 | A225 A235 A230 A236 | A240 A230 A228 | A225 A228 A230 A240 | A237 A230 A238 A225 | A225 A238 A237 | A235 A225 A226 | A225 A226 A230 A235 | A230 A235 A236 | A233 A230 A236 A225 | A225 A234 A230 A233 | A238 A230 A227 A225 | A225 A227 A238 | A237 A230 A238 | A234 A225 A237 A230 | A230 A226 A235 | A236 A230 A235 A225 | A238 A230 A227 | A237 A225 A238 A230 | A225 A235 A230 A226 | A227 A230 A238 A225
fillet "フィレット1" radius 2 8 edges at (-8.8605, 20.2737, 3.75) (-11.4328, 16.4987, 3.75) (-9.9333, 8.5848, 3.75) (-6.1583, 6.0125, 3.75) (1.7555, 7.512, 3.75) (4.3279, 11.287, 3.75) (2.8283, 19.2009, 3.75) (-0.9467, 21.7732, 3.75)
extrude "押し出し3" cut sketch "スケッチ1" along normal blind 0.8 contours A232 A225 A241 | A225 A241 A230 A232 | A231 A230 A239 A225 | A225 A239 A231 | A241 A225 A242 | A225 A242 A230 A241 | A232 A230 A241 A225 | A230 A241 A232 | A239 A230 A240 A225 | A225 A240 A239 | A231 A230 A239 | A225 A239 A230 A231 | A242 A225 A229 | A225 A229 A230 A242 | A241 A230 A242 A225 | A230 A242 A241 | A233 A225 A236 | A225 A236 A230 A233 | A240 A230 A228 A225 | A225 A228 A240 | A239 A230 A240 | A225 A240 A230 A239 | A234 A230 A237 A225 | A225 A237 A234 | A229 A225 | A225 A229 A230 | A242 A230 A229 A225 | A230 A229 A242 | A236 A225 A235 | A225 A235 A230 A236 | A230 A236 A233 | A228 A230 A225 | A225 A228 | A240 A230 A228 | A225 A228 A230 A240 | A237 A230 A238 A225 | A225 A238 A237 | A234 A230 A237 | A230 A229 | A235 A225 A226 | A225 A226 A230 A235 | A230 A235 A236 | A233 A230 A236 A225 | A228 A230 | A238 A230 A227 A225 | A225 A227 A238 | A237 A230 A238 | A234 A225 A237 A230 | A226 A225 | A225 A226 A230 | A230 A226 A235 | A236 A230 A235 A225 | A227 A230 A225 | A225 A227 | A238 A230 A227 | A237 A225 A238 A230 | A225 A235 A230 A226 | A230 A226 | A227 A230 A238 A225 | A227 A230
